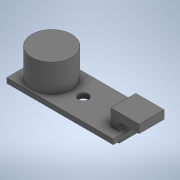
# Autodesk Inventor part: Buzzer
Saved by Autodesk Inventor 2020 (Build 240168000, 168)
## iProperties
Created: 2020-01-01
Part Number: Buzzer
Material: Argent
Document SubType Name: Modeling
Designer: Manuel Enzo
Density: 10.49 g/cm^3
Appearance: Gris
Author: Manuel Enzo
Autodesk Inventor part; units mm, degrees
ref_plane "YZ Plane" through (0, 0, 0) normal (1, 0, 0) x (0, 1, 0)
ref_plane "XZ Plane" through (0, 0, 0) normal (0, 1, 0) x (-1, 0, 0)
ref_plane "XY Plane" through (0, 0, 0) normal (0, 0, 1) x (1, 0, 0)
sketch "Esquisse1" plane through (0, 0, 0) normal (0, 1, 0) x (-1, 0, 0)
  line L0 (0, 0) -> (32, 0)
  line L1 (32, 0) -> (32, -13)
  line L2 (32, -13) -> (0, -13)
  line L3 (0, -13) -> (0, 0)
  circle A0 centre (25, -6.5) radius 6
  line L4 (3.5, -2.75) -> (1, -2.75)
  line L5 (1, -2.75) -> (1, -10.25)
  line L6 (1, -10.25) -> (3.5, -10.25)
  line L7 (3.5, -10.25) -> (3.5, -2.75)
  circle A1 centre (15.5, -6.5) radius 2.5
  circle A2 centre (15.5, -6.5) radius 1.5
  dimension "d0" = 13
  dimension "d1" = 32
  dimension "d2" = 12
  dimension "d3" = 7
  dimension "d4" = 7.5
  dimension "d5" = 1
  dimension "d6" = 2.5
  dimension "d7" = 2.75
  dimension "d8" = 2.75
  dimension "d9" = 5
  dimension "d10" = 9.5
  dimension "d11" = 6.5
  dimension "d12" = 6.5
  dimension "d13" = 1
  constraints: 16 end point, 4 parallel, 3 centre point, 2 horizontal, 2 perpendicular, 1 coincident
  measures "d0" distance between parallel lines of L0 L2
  measures "d1" distance between parallel lines of L3 L1
  measures "d2" diameter of A0
  measures "d3" distance from line of L1 A0.centre
  measures "d4" distance between parallel lines of L4 L6
  measures "d5" distance between parallel lines of L3 L5
  measures "d6" distance between parallel lines of L5 L7
  measures "d7" distance between parallel lines of L0 L4
  measures "d8" distance between parallel lines of L2 L6
  measures "d9" diameter of A1
  measures "d10" distance of A1.centre A0.centre
  measures "d11" distance from line of L0 A1.centre
  measures "d12" distance from line of L2 A0.centre
  measures "d13" radial gap between concentric circles of A1 A2
extrude "Extrusion1" add sketch "Esquisse1" along normal blind 1.5 contours L0 L1 L2 L3 | A1
extrude "Extrusion2" add sketch "Esquisse1" along normal blind 10 contours A0
extrude "Extrusion3" add sketch "Esquisse1" along normal blind 6.5 contours L7 L6 L5 L4
sketch "Esquisse2" plane through (-1, 1.5, -10.25) normal (1, 0, 0) x (0, 0, -1)
  line L0 (-7.5, 0) -> (-7.5, 5) projected
  line L1 (0, 0) -> (0, 5) projected
  line L2 (-7.5, 5) -> (0, 5)
  line L3 (0, 5) -> (0, 2.5)
  line L4 (0, 2.5) -> (-7.5, 2.5)
  line L5 (-7.5, 2.5) -> (-7.5, 5)
  point P0 (-10.25, -1.5)
  point P1 (-7.5, 2.5)
  dimension "d20" = 2.5
  constraints: 8 end point, 2 parallel, 1 horizontal, 1 midpoint, 1 perpendicular
  measures "d20" distance between parallel lines of L2 L4
extrude "Extrusion4" add sketch "Esquisse2" along normal blind 6
extrude "Extrusion5" add sketch "Esquisse1" against normal blind 1.5 contours L7 L6 L5 L4
